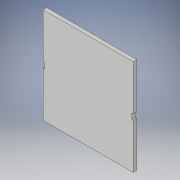
# Autodesk Inventor part: Middle Platform
Saved by Autodesk Inventor 2018 (Build 220112000, 112)
## iProperties
Created: 2019-01-10
Part Number: Middle Platform
Material: Generic
Document SubType Name: Modeling
Designer: maste
Density: 1 g/cm^3
Appearance: Default
Author: maste
Autodesk Inventor part; units mm, degrees
ref_plane "YZ Plane" through (0, 0, 0) normal (1, 0, 0) x (0, 1, 0)
ref_plane "XZ Plane" through (0, 0, 0) normal (0, 1, 0) x (-1, 0, 0)
ref_plane "XY Plane" through (0, 0, 0) normal (0, 0, 1) x (1, 0, 0)
sketch "Sketch1" plane through (0, 0, 0) normal (0, 0, 1) x (1, 0, 0)
  line L0 (0, 0) -> (622.8588, 0)
  line L1 (622.8588, 0) -> (622.8588, 662.5844)
  line L2 (622.8588, 662.5844) -> (0, 662.5844)
  line L3 (0, 662.5844) -> (0, 0)
  line L4 (622.8588, 331.2922) -> (622.8588, 351.2947)
  line L5 (622.8588, 351.2947) -> (622.8588, 311.2897)
  line L6 (622.8588, 351.2947) -> (613.4862, 351.2947)
  line L7 (613.4862, 351.2947) -> (613.4862, 311.2897)
  line L8 (613.4862, 311.2897) -> (622.8588, 311.2897)
  line L9 (622.8588, 311.2897) -> (622.8588, 351.2947)
  line L10 (0, 351.2947) -> (9.3726, 351.2947)
  line L11 (9.3726, 351.2947) -> (9.3726, 311.2897)
  line L12 (9.3726, 311.2897) -> (0, 311.2897)
  line L13 (0, 311.2897) -> (9.3726, 311.2897)
  line L14 (9.3726, 311.2897) -> (9.3726, 351.2947)
  line L15 (9.3726, 351.2947) -> (0, 351.2947)
  line L16 (0, 351.2947) -> (0, 311.2897)
  dimension "d0" = 622.8588
  dimension "d1" = 662.5844
  dimension "d2" = 20.0025
  dimension "d3" = 40.005
  dimension "d4" = 9.3726
  constraints: 34 end point, 6 parallel, 3 horizontal, 3 perpendicular, 2 point on line, 1 midpoint
  measures "d0" distance of L2.end L1.end
  measures "d1" distance of L1.end L0.end
  measures "d2" distance of L4.start L4.end
  measures "d3" distance of L4.end L5.end
  measures "d4" distance of L8.end L7.end
extrude "Extrusion1" add sketch "Sketch1" along normal blind 25.4 contours L3 L12 L11 L10 L2 L1 L6 L7 L8 L0
body "Solid1"
